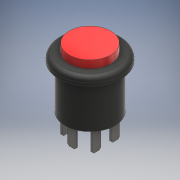
# Autodesk Inventor part: switch
Saved by Autodesk Inventor 2018 (Build 220112000, 112)
## iProperties
Created: 2019-03-10
Part Number: switch
Material: 一般
Document SubType Name: Modeling
Designer: ku_sk
Density: 1 g/cm^3
Appearance: 滑らか - 黒
Author: ku_sk
Autodesk Inventor part; units mm, degrees
ref_plane "YZ Plane" through (0, 0, 0) normal (1, 0, 0) x (0, 1, 0)
ref_plane "XZ Plane" through (0, 0, 0) normal (0, 1, 0) x (-1, 0, 0)
ref_plane "XY Plane" through (0, 0, 0) normal (0, 0, 1) x (1, 0, 0)
sketch "スケッチ1" plane through (0, 0, 0) normal (0, 0, 1) x (1, 0, 0)
  circle A0 centre (0, 0) radius 8
  dimension "d0" = 16
  constraints: 1 centre point, 1 coincident
  measures "d0" diameter of A0
extrude "押し出し1" add sketch "スケッチ1" along normal blind 14
sketch "スケッチ2" plane through (0, 0, 14) normal (0, 0, 1) x (1, 0, 0)
  circle A0 centre (0, 0) radius 10
  dimension "d3" = 20
  constraints: 1 centre point, 1 coincident
  measures "d3" diameter of A0
extrude "押し出し2" add sketch "スケッチ2" along normal blind 2.5
fillet "フィレット1" radius 1.5 1 edges at (-10, 0, 16.5)
sketch "スケッチ3" plane through (0, 0, 16.5) normal (0, 0, 1) x (1, 0, 0)
  circle A0 centre (0, 0) radius 6.665
  dimension "d7" = 13.33
  constraints: 1 centre point, 1 coincident
  measures "d7" diameter of A0
extrude "押し出し3" add sketch "スケッチ3" along normal blind 2.5
sketch "スケッチ4" plane through (0, 0, 0) normal (0, 0, -1) x (-1, 0, 0)
  line L0 (-1.35, 5.83) -> (1.35, 5.83)
  line L1 (1.35, 5.83) -> (1.35, 5.33)
  line L2 (1.35, 5.33) -> (-1.35, 5.33)
  line L3 (-1.35, 5.33) -> (-1.35, 5.83)
  line L4 (0, -14) -> (0, 14) projected
  line L5 (14, 0) -> (-14, 0) projected
  line L6 (-1.35, -5.83) -> (1.35, -5.83)
  line L7 (1.35, -5.83) -> (1.35, -5.33)
  line L8 (1.35, -5.33) -> (-1.35, -5.33)
  line L9 (-1.35, -5.33) -> (-1.35, -5.83)
  line L10 (4.6, 4.36) -> (5.1, 4.36)
  line L11 (5.1, 4.36) -> (5.1, 1.66)
  line L12 (5.1, 1.66) -> (4.6, 1.66)
  line L13 (4.6, 1.66) -> (4.6, 4.36)
  line L14 (4.6, -4.36) -> (5.1, -4.36)
  line L15 (5.1, -4.36) -> (5.1, -1.66)
  line L16 (5.1, -1.66) -> (4.6, -1.66)
  line L17 (4.6, -1.66) -> (4.6, -4.36)
  line L18 (-4.6, 4.36) -> (-5.1, 4.36)
  line L19 (-5.1, 4.36) -> (-5.1, 1.66)
  line L20 (-5.1, 1.66) -> (-4.6, 1.66)
  line L21 (-4.6, 1.66) -> (-4.6, 4.36)
  line L22 (-4.6, -1.66) -> (-4.6, -4.36)
  line L23 (-4.6, -4.36) -> (-5.1, -4.36)
  line L24 (-5.1, -4.36) -> (-5.1, -1.66)
  line L25 (-5.1, -1.66) -> (-4.6, -1.66)
  point P0 (0, 0)
  point P1 (0, 5.83)
  point P2 (0, -5.83)
  dimension "d10" = 2.7
  dimension "d11" = 5.83
  dimension "d12" = 0.5
  dimension "d13" = 2.7
  dimension "d14" = 0.5
  dimension "d15" = 4.36
  dimension "d16" = 5.1
  constraints: 48 end point, 17 symmetric about line, 4 parallel, 2 horizontal, 2 perpendicular, 1 midpoint, 1 point on line
  measures "d10" distance of L0.start L0.end
  measures "d11" distance from line of point (0, 0) L0
  measures "d12" distance between parallel lines of L0 L2
  measures "d13" distance of L10.end L11.end
  measures "d14" distance between parallel lines of L13 L11
  measures "d15" distance between parallel lines of L5 L10
  measures "d16" distance between parallel lines of L4 L11
extrude "押し出し4" add sketch "スケッチ4" along normal blind 7.16
chamfer "面取り1" distance 0.5 angle 45 12 edges at (-4.85, -4.36, -7.16) (-4.85, -1.66, -7.16) (-4.85, 1.66, -7.16) (-4.85, 4.36, -7.16) (-1.35, 5.58, -7.16) (1.35, 5.58, -7.16) (4.85, 4.36, -7.16) (4.85, 1.66, -7.16) (4.85, -1.66, -7.16) (4.85, -4.36, -7.16) (1.35, -5.58, -7.16) (-1.35, -5.58, -7.16)
equation "\"d13\" = d10"
equation "\"d14\" = d12"
